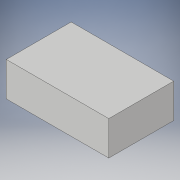
# Autodesk Inventor part: Block
Saved by Autodesk Inventor 2019 (Build 230136000, 136)
## iProperties
Created: 2021-12-15
Part Number: Block
Material: Generisch
Document SubType Name: Modeling
Designer: Bergi
Density: 1 g/cm^3
Appearance: Vorgabe
Author: Bergi
Autodesk Inventor part; units mm, degrees
ref_plane "YZ Plane" through (0, 0, 0) normal (1, 0, 0) x (0, 1, 0)
ref_plane "XZ Plane" through (0, 0, 0) normal (0, 1, 0) x (-1, 0, 0)
ref_plane "XY Plane" through (0, 0, 0) normal (0, 0, 1) x (1, 0, 0)
sketch "Skizze1" plane through (0, 0, 0) normal (0, 1, 0) x (-1, 0, 0)
  line L0 (-7.5, 4.75) -> (7.5, 4.75)
  line L1 (7.5, 4.75) -> (7.5, -4.75)
  line L2 (7.5, -4.75) -> (-7.5, -4.75)
  line L3 (-7.5, -4.75) -> (-7.5, 4.75)
  line L4 (-7.5, 4.75) -> (7.5, -4.75) construction
  line L5 (7.5, 4.75) -> (-7.5, -4.75) construction
  point P0 (0, 0)
  dimension "d0" = 15
  dimension "d1" = 9.5
  constraints: 12 end point, 2 midpoint, 2 parallel, 1 horizontal, 1 perpendicular
  measures "d0" distance of L1.end L2.end
  measures "d1" distance of L0.end L1.end
extrude "Extrusion1" add sketch "Skizze1" along normal blind 5
